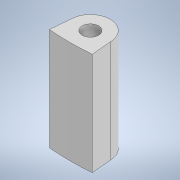
# Autodesk Inventor part: Spacer
Saved by Autodesk Inventor 2020.1 (Build 241239000, 239)
## iProperties
Created: 2022-03-19
Part Number: Spacer
Material: Generic
Document SubType Name: Modeling
Designer: OEM
Density: 1 g/cm^3
Appearance: Default
Author: OEM
Autodesk Inventor part; units mm, degrees
ref_plane "YZ Plane" through (0, 0, 0) normal (1, 0, 0) x (0, 1, 0)
ref_plane "XZ Plane" through (0, 0, 0) normal (0, 1, 0) x (-1, 0, 0)
ref_plane "XY Plane" through (0, 0, 0) normal (0, 0, 1) x (1, 0, 0)
sketch "Sketch1" plane through (0, 0, 0) normal (0, 1, 0) x (-1, 0, 0)
  circle A0 centre (0, 0) radius 60 construction
  circle A1 centre (0, 0) radius 55 construction
  circle A2 centre (0, 55) radius 2
  arc A3 (5.2293, 59.7717) -> (-5.2293, 59.7717) centre (0, 0) ccw
  line L0 (0, 0) -> (5.2293, 59.7717) construction
  line L1 (0, 0) -> (60, 0) construction
  line L2 (0, 0) -> (-5.2293, 59.7717) construction
  line L3 (0, 24.4692) -> (0, -19) construction
  arc A4 (-4.7936, 54.7907) -> (4.7936, 54.7907) centre (0, 55) ccw
  line L4 (4.7936, 54.7907) -> (5.2293, 59.7717)
  line L5 (-5.2293, 59.7717) -> (-4.7936, 54.7907)
  dimension "d0" = 120
  dimension "d1" = 110
  dimension "d2" = 4
  dimension "d4" = 10
  dimension "d5" = 5
  constraints: 12 end point, 7 point on circle, 4 centre point, 4 coincident, 2 point on line, 1 collinear, 1 equal length, 1 horizontal, 1 vertical, 3 other
  measures "d1" diameter of A1
  measures "d2" diameter of A2
  measures "d4" angle of L0 L2
  measures "d5" angle of L3 L0
extrude "Extrusion1" add sketch "Sketch1" along normal blind 25
equation "\"d5\" = 0.5 * d4"
body "Solid1"
